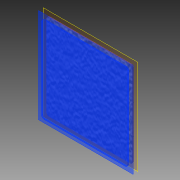
# Autodesk Inventor part: piastra_superiorissima
Saved by Autodesk Inventor 2014 SP1 (Build 180222100, 222)
## iProperties
Created: 2015-04-08
Part Number: piastra_superiorissima
Material: Generic
Document SubType Name: Modeling
Designer: Giorgio Nuzzo
Density: 1 g/cm^3
Appearance: Cherry - Natural Low Gloss
Author: Giorgio Nuzzo
Autodesk Inventor part; units mm, degrees
ref_plane "YZ Plane" through (0, 0, 0) normal (1, 0, 0) x (0, 1, 0)
ref_plane "XZ Plane" through (0, 0, 0) normal (0, 1, 0) x (-1, 0, 0)
ref_plane "XY Plane" through (0, 0, 0) normal (0, 0, 1) x (1, 0, 0)
ref_plane "Work Plane1" through (-0.0001, 0, 0) normal (0, -1, 0) x (-1, 0, 0)
sketch "Sketch1" plane through (-0.0001, 0, 0) normal (0, -1, 0) x (-1, 0, 0)
  circle A0 centre (-100.5001, -100.5001) radius 1.6 construction
  circle A1 centre (-100.5001, 100.5001) radius 1.6 construction
  circle A2 centre (100.5001, 100.5001) radius 1.6 construction
  circle A3 centre (100.5001, -100.5001) radius 1.6 construction
  line L0 (-97.4996, 3.9999) -> (-97.4996, 82.5416) construction
  line L1 (-97.4996, 82.5416) -> (-72.0063, 57.0482) construction
  line L2 (-72.0063, 57.0482) -> (-72.0063, 3.9999) construction
  line L3 (-72.0063, 3.9999) -> (-97.4996, 3.9999) construction
  line L4 (-97.4996, -82.5021) -> (-97.4996, -4.0001) construction
  line L5 (-97.4996, -4.0001) -> (-72.0063, -4.0001) construction
  line L6 (-72.0063, -4.0001) -> (-72.0063, -57.0088) construction
  line L7 (-72.0063, -57.0088) -> (-97.4996, -82.5021) construction
  line L8 (97.4891, -4.0001) -> (97.4891, -82.4901) construction
  line L9 (97.4891, -82.4901) -> (72.0063, -57.007) construction
  line L10 (72.0063, -57.007) -> (72.0063, -4.0001) construction
  line L11 (72.0063, -4.0001) -> (97.4891, -4.0001) construction
  line L12 (97.4891, 82.4918) -> (97.4891, 4.0106) construction
  line L13 (97.4891, 4.0106) -> (72.0063, 3.9999) construction
  line L14 (72.0063, 3.9999) -> (72.0063, 57.0089) construction
  line L15 (72.0063, 57.0089) -> (97.4891, 82.4918) construction
  line L16 (3.998, 18.9804) -> (3.998, 93.318) construction
  line L17 (3.998, 93.318) -> (41.1668, 56.1492) construction
  line L18 (41.1668, 56.1492) -> (3.998, 18.9804) construction
  line L19 (41.1668, -56.0334) -> (3.998, -93.2022) construction
  line L20 (3.998, -93.2022) -> (3.998, -18.8647) construction
  line L21 (3.998, -18.8647) -> (41.1668, -56.0334) construction
  line L22 (-4.0018, -18.9081) -> (-4.0018, -93.1785) construction
  line L23 (-4.0018, -93.1785) -> (-41.1372, -56.0431) construction
  line L24 (-41.1372, -56.0431) -> (-4.0018, -18.9081) construction
  line L25 (-4.0018, 93.294) -> (-4.0018, 19.0236) construction
  line L26 (-4.0018, 19.0236) -> (-41.1372, 56.1588) construction
  line L27 (-41.1372, 56.1588) -> (-4.0018, 93.294) construction
  line L28 (45.4095, 60.3918) -> (8.292, 97.5093) construction
  line L29 (8.292, 97.5093) -> (82.5267, 97.5093) construction
  line L30 (82.5267, 97.5093) -> (45.4095, 60.3918) construction
  line L31 (8.292, -97.3935) -> (45.4095, -60.2762) construction
  line L32 (45.4095, -60.2762) -> (82.5267, -97.3935) construction
  line L33 (82.5267, -97.3935) -> (8.292, -97.3935) construction
  line L34 (-8.272, -97.3935) -> (-82.4876, -97.3935) construction
  line L35 (-82.4876, -97.3935) -> (-45.3798, -60.2857) construction
  line L36 (-45.3798, -60.2857) -> (-8.272, -97.3935) construction
  line L37 (-8.272, 97.5093) -> (-45.3798, 60.4015) construction
  line L38 (-45.3798, 60.4015) -> (-82.4876, 97.5093) construction
  line L39 (-82.4876, 97.5093) -> (-8.272, 97.5093) construction
  line L40 (-50.0062, -35.0087) -> (-50.0062, 35.0482) construction
  line L41 (-50.0062, 35.0482) -> (-19.4004, 4.4423) construction
  line L42 (-19.4004, 4.4423) -> (-19.4004, -4.4028) construction
  line L43 (-19.4004, -4.4028) -> (-50.0062, -35.0087) construction
  line L44 (19.4508, -4.4518) -> (19.4508, 4.4535) construction
  line L45 (19.4508, 4.4535) -> (50.0062, 35.0089) construction
  line L46 (50.0062, 35.0089) -> (50.0062, -35.007) construction
  line L47 (50.0062, -35.007) -> (19.4508, -4.4518) construction
  line L48 (101.5001, -107.5001) -> (-101.5001, -107.5001) projected
  arc A4 (101.5001, -107.5001) -> (107.5001, -101.5001) centre (101.5001, -101.5001) ccw projected
  line L49 (107.5001, 101.5001) -> (107.5001, -101.5001) projected
  arc A5 (107.5001, 101.5001) -> (101.5001, 107.5001) centre (101.5001, 101.5001) ccw projected
  line L50 (-101.5001, 107.5001) -> (101.5001, 107.5001) projected
  arc A6 (-101.5001, 107.5001) -> (-107.5001, 101.5001) centre (-101.5001, 101.5001) ccw projected
  line L51 (-107.5001, -101.5001) -> (-107.5001, 101.5001) projected
  arc A7 (-107.5001, -101.5001) -> (-101.5001, -107.5001) centre (-101.5001, -101.5001) ccw projected
extrude "Extrusion1" add sketch "Sketch1" along normal blind 3
body "Solid1"
